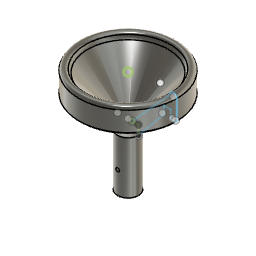
Nozzle and Funnel V.1 v5 (Autodesk Fusion 360 design; units mm, degrees)
Autodesk Fusion 360 part; units mm, degrees
sketch "Sketch1" plane through (0, 0, 0) normal (0, 1, 0) x (1, 0, 0)
  line L0 (3, -44) -> (7.49, -44)
  line L1 (7.49, -44) -> (7.49, 0)
  line L2 (7.49, 0) -> (3.05, 0)
  line L3 (3.05, 0) -> (3.05, -35.1225)
  line L4 (3.05, -35.1225) -> (1, -30.1)
  line L5 (1, -35) -> (3, -44)
  spline S0 degree 2 poles (1, -35) (0.2804, -31.7616) (1, -30.1) knots 0 0 0 0.50243 0.50243 0.50243 weights 1 3 1
  point P0 (0, -44)
  point P1 (7.49, -44)
  point P2 (7.49, -44)
  point P3 (7.49, 0)
  point P4 (3.05, 0)
  point P5 (1, -30.1)
  point P6 (3, -44)
  point P7 (1, -35)
  dimension "d1" = 44
  dimension "d2" = 44
  dimension "d3" = 44
  dimension "d4" = 7.49
  dimension "d5" = 7.49
  dimension "d6" = 3.05
  dimension "d7" = 3
  dimension "d9" = 13.9
  dimension "d10" = 9
  dimension "d11" = 1
  dimension "d12" = 1
  constraint coincident P6 L0.start
  constraint coincident P2 P1
  constraint coincident P3 L1.end
  constraint vertical L1
  constraint coincident P4 L2.end
  constraint perpendicular L1 L2
  constraint perpendicular L2 L3
  constraint coincident P5 L4.end
  constraint coincident P7 L5.start
  measures "d1" distance of origin P0
  measures "d2" vertical distance of P2 L1.end
  measures "d3" distance of P2 P3
  measures "d4" distance of origin P3
  measures "d5" distance of P0 P1
  measures "d6" distance of origin P4
  measures "d7" horizontal distance of P0 P6
  measures "d9" vertical distance of P0 P5
  measures "d10" vertical distance of P0 P7
  measures "d11" horizontal distance of P0 P5
  measures "d12" horizontal distance of P0 P7
revolve "Revolve1" add sketch "Sketch1" angle 360 about axis through (0, 0, 1.75) along (0, 0, 1) makes body 1
hole "Hole1" at (0, -7.49, 15.9907) direction (0, 1, 0) diameter 2.5 end through all bodies 1
copy_body "Body->Comp1" bodies 1 removing the originals makes body 2 in component "Component"
sketch "Sketch1 (2)" plane through (0, 0, 0) normal (0, 1, 0) x (1, 0, 0) in component "Nozzle"
  line L0 (3, -44) -> (28.8955, -72.6)
  line L1 (7.51, -37.3714) -> (7.51, -44)
  line L2 (7.51, -44) -> (3, -44)
  line L3 (35, -74) -> (35, -60)
  line L4 (34, -59) -> (31.586, -59)
  line L5 (30.586, -60) -> (30.586, -65)
  line L6 (30.586, -65) -> (25.698, -65)
  line L7 (25.698, -65) -> (25.698, -59.7807)
  line L8 (25.4694, -59.1444) -> (7.51, -37.3714)
  arc A0 (30.3385, -74.9042) -> (35, -74) centre (32.5816, -74) ccw
  arc A1 (31.586, -59) -> (30.586, -60) centre (31.586, -60) ccw
  arc A2 (35, -60) -> (34, -59) centre (34, -60) ccw
  arc A3 (25.698, -59.7807) -> (25.4694, -59.1444) centre (24.698, -59.7807) ccw
  arc A4 (30.3385, -74.9042) -> (28.8955, -72.6) centre (23.1505, -77.8017) ccw
  point P0 (0, -44)
  point P1 (7.51, -44)
  point P2 (-7.5, -44)
  point P3 (3, -44)
  point P4 (0, -73)
  point P5 (7.51, -37.3714)
  dimension "d17" = 7.51
  dimension "d20" = 35
  dimension "d21" = 25.698
  dimension "d22" = 30.586
  dimension "d23" = 8
  dimension "d24" = 1
  dimension "d25" = 7.75
  dimension "d26" = 44.3874
  constraint coincident P3 L0.start
  constraint coincident P5 L1.start
  constraint coincident P1 L1.end
  constraint perpendicular L1 L2
  constraint coincident L3.start A0.end
  constraint perpendicular L3 L4
  constraint perpendicular L4 L5
  constraint perpendicular L5 L6
  constraint perpendicular L6 L7
  constraint tangent L4 A1
  constraint tangent L5 A1
  constraint tangent L3 A2
  constraint tangent L4 A2
  constraint equal A1 A2
  constraint tangent L7 A3
  constraint tangent L8 A3
  constraint equal A1 A3
  constraint tangent A0 A4
  constraint tangent L0 A4
  measures "d17" distance of P0 L1.end
  measures "d20" horizontal distance of P4 L3.start
  measures "d21" horizontal distance of P4 L6.end
  measures "d22" horizontal distance of P4 L5.end
  measures "d23" vertical distance of P4 L6.end
  measures "d24" radius of A1
  measures "d25" radius of A4
  measures "d26" distance of P5 A0.centre
revolve "Revolve1'" add sketch "Sketch1 (2)" angle 360 about axis through (0, 0, 44) along (0, 0, -1) separate body makes body 3 in component "Nozzle"
sketch "Sketch1 (3)" plane through (0, 0, 0) normal (0, 0, 1) x (1, 0, 0) in component "Body V1.0"
  circle A0 centre (0, 0) radius 25.4951
  circle A1 centre (0, 0) radius 30.4138
  constraint coincident A0.centre A1.centre
  constraint concentric A0 A1
extrude "Extrude1" add sketch "Sketch1 (3)" along normal up to surface (65 mm away) and the other way blind 100 separate body makes body 4 in component "Body V1.0"
sketch "Sketch2" plane through (0, 0, -100) normal (0, 0, -1) x (1, 0, 0) in component "Body V1.0"
  circle A0 centre (0, 0) radius 25.4951
  circle A1 centre (0, 0) radius 30.4138
  circle A2 centre (0, 0) radius 30.4138
  constraint concentric A0 A2
extrude "Extrude2" add sketch "Sketch2" against normal blind 5 contours A0 bodies 4 in component "Body V1.0"
hole "Hole1'" at (0, -30.4138, -46.6912) direction (0, 1, 0) diameter 20 depth 20 tip angle 180 bodies 4 in component "Body V1.0"
component "Nozzle" placed x (1, 0, 0) y (0, 1, 0) z (0, 0, 1) at (0, 0, 0)
component "Component" placed x (1, 0, 0) y (0, 1, 0) z (0, 0, 1) at (0, 0, 0)
component "Body V1.0" placed x (1, 0, 0) y (0, 1, 0) z (0, 0, 1) at (0, 0, 0)
component "Component'" placed x (1, 0, 0) y (0, 1, 0) z (0, 0, 1) at (0, 0, 0) in component "Body V1.0"
